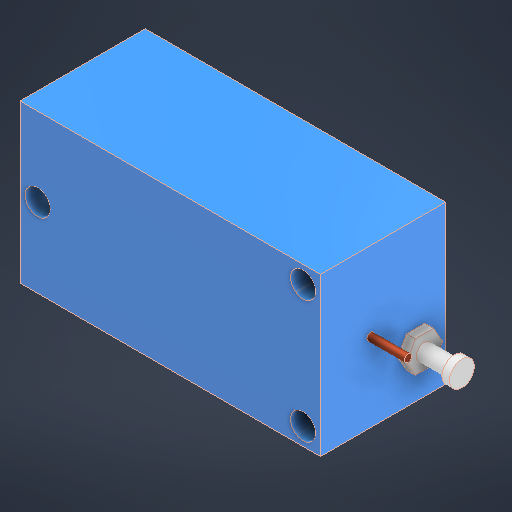
# Autodesk Inventor part: BTBody
Saved by Autodesk Inventor 2026.2 (Build 302298010, 298A)
## iProperties
Created: 2026-06-12
Part Number: BTBody
Material: Generic
Document SubType Name: Modeling
Designer: sonata
Density: 1 g/cm^3
Appearance: Default
Author: sonata
Autodesk Inventor part; units mm, degrees
ref_plane "YZ Plane" through (0, 0, 0) normal (1, 0, 0) x (0, 1, 0)
ref_plane "XZ Plane" through (0, 0, 0) normal (0, 1, 0) x (-1, 0, 0)
ref_plane "XY Plane" through (0, 0, 0) normal (0, 0, 1) x (1, 0, 0)
sketch "Sketch1" plane through (0, 0, 0) normal (0, 0, 1) x (1, 0, 0)
  line L0 (0, 0) -> (30.48, 0)
  line L1 (30.48, 0) -> (30.48, 16.002)
  line L2 (30.48, 16.002) -> (0, 16.002)
  line L3 (0, 16.002) -> (0, 0)
  dimension "d0" = 30.48
  dimension "d1" = 16.002
  constraints: 8 end point, 2 parallel, 1 horizontal, 1 perpendicular
  measures "d0" distance of L1.end L2.end
  measures "d1" distance of L0.end L1.end
extrude "Extrusion1" add sketch "Sketch1" along normal blind 12.7
sketch "Sketch2" plane through (0, 0, 12.7) normal (0, 0, 1) x (1, 0, 0)
  line L0 (0, 0) -> (30.48, 0) projected
  line L1 (0, 16.002) -> (0, 0) projected
  point P0 (1.778, 8.001)
  point P1 (28.702, 14.224)
  point P2 (28.702, 1.778)
  dimension "d4" = 26.924
  dimension "d5" = 8.001
  dimension "d6" = 1.778
  dimension "d7" = 1.778
  dimension "d8" = 12.446
  constraints: 1 vertical alignment
  measures "d4" horizontal distance of point (1.778, 8.001) point (28.702, 1.778)
  measures "d5" distance from line of point (1.778, 8.001) L0
  measures "d6" distance from line of point (1.778, 8.001) L1
  measures "d7" distance from line of point (28.702, 1.778) L0
  measures "d8" distance of point (28.702, 1.778) point (28.702, 14.224)
hole "Hole1" at (1.778, 8.001, 12.7) at (28.702, 14.224, 12.7) at (28.702, 1.778, 12.7) direction (0, 0, -1) diameter 2.54 end through all
sketch "Sketch3" plane through (30.48, 0, 0) normal (1, 0, 0) x (0, 0, -1)
  circle A0 centre (-7.62, 8.001) radius 0.381
  line L0 (-12.7, 0) -> (-12.7, 16.002) projected
  line L1 (0, 0) -> (-12.7, 0) projected
  dimension "d17" = 0.762
  dimension "d18" = 5.08
  dimension "d19" = 8.001
  constraints: 1 centre point
  measures "d17" diameter of A0
  measures "d18" distance from line of L0 A0.centre
  measures "d19" distance from line of A0.centre L1
extrude "Extrusion2" add sketch "Sketch3" along normal blind 3.81
sketch "Sketch4" plane through (30.48, 0, 0) normal (1, 0, 0) x (0, 0, -1)
  line L0 (-4.8958, 4.826) -> (-3.9719, 6.4262)
  line L1 (-3.9719, 6.4262) -> (-2.1241, 6.4262)
  line L2 (-2.1241, 6.4262) -> (-1.2002, 4.826)
  line L3 (-1.2002, 4.826) -> (-2.1241, 3.2258)
  line L4 (-2.1241, 3.2258) -> (-3.9719, 3.2258)
  line L5 (-3.9719, 3.2258) -> (-4.8958, 4.826)
  line L6 (-3.9719, 3.2258) -> (-2.1241, 6.4262) construction
  line L7 (-2.1241, 3.2258) -> (-3.9719, 6.4262) construction
  line L8 (-12.7, 0) -> (-12.7, 16.002) projected
  line L9 (0, 0) -> (-12.7, 0) projected
  point P0 (-3.048, 4.826)
  point P1 (-3.048, 4.826)
  dimension "d22" = 120
  dimension "d23" = 9.652
  dimension "d24" = 4.826
  dimension "d25" = 3.2004
  constraints: 16 end point, 5 equal length, 2 midpoint, 2 vertical alignment, 1 horizontal, 1 horizontal alignment
  measures "d22" angle of L0 L5
  measures "d23" distance from line of point (-3.048, 4.826) L8
  measures "d24" distance from line of point (-3.048, 4.826) L9
  measures "d25" distance between parallel lines of L1 L4
extrude "Extrusion3" add sketch "Sketch4" along normal blind 0.889
sketch "Sketch5" plane through (31.369, 0, 0) normal (1, 0, 0) x (0, 0, -1)
  line L0 (-3.9719, 3.2258) -> (-2.1241, 3.2258) projected
  line L1 (-1.2002, 4.826) -> (-2.1241, 6.4262) projected
  line L2 (-3.9719, 3.2258) -> (-2.1241, 6.4262)
  line L3 (-1.2002, 4.826) -> (-4.8958, 4.826)
  circle A0 centre (-3.048, 4.826) radius 0.8255
  point P0 (0, 0)
  dimension "d28" = 1.651
  constraints: 4 end point, 1 centre point, 1 midpoint
  measures "d28" diameter of A0
extrude "Extrusion4" add sketch "Sketch5" along normal blind 3.048 contours A0 L2 L3 | L3 L2 A0 | L2 L3 A0 | L2 A0 L3
sketch "Sketch6" plane through (34.417, 4.826, 3.048) normal (1, 0, 0) x (0, 0, -1)
  circle A0 centre (0, 0) radius 1.27
  circle A1 centre (0, 0) radius 0.8255 projected
  point P0 (3.048, -4.826)
  dimension "d31" = 2.54
  constraints: 1 centre point, 1 concentric
  measures "d31" diameter of A0
extrude "Extrusion5" add sketch "Sketch6" along normal blind 0.762 contours A0 | A1
body "Solid1"
